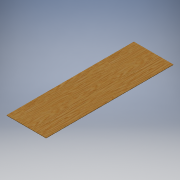
# Autodesk Inventor part: Table top
Saved by Autodesk Inventor 2019.4 (Build 234330000, 330)
## iProperties
Created: 2020-02-27
Part Number: Table top
Material: Plywood, Finish
Document SubType Name: Modeling
Designer: admin
Density: 0.552 g/cm^3
Appearance: Plywood - New
Author: admin
Autodesk Inventor part; units mm, degrees
ref_plane "YZ Plane" through (0, 0, 0) normal (1, 0, 0) x (0, 1, 0)
ref_plane "XZ Plane" through (0, 0, 0) normal (0, 1, 0) x (-1, 0, 0)
ref_plane "XY Plane" through (0, 0, 0) normal (0, 0, 1) x (1, 0, 0)
sketch "Sketch1" plane through (0, 0, 0) normal (0, 1, 0) x (-1, 0, 0)
  line L0 (-225, 725) -> (225, 725)
  line L1 (225, 725) -> (225, -725)
  line L2 (225, -725) -> (-225, -725)
  line L3 (-225, -725) -> (-225, 725)
  line L4 (-225, 725) -> (225, -725) construction
  line L5 (225, 725) -> (-225, -725) construction
  point P0 (0, 0)
  dimension "d0" = 450
  dimension "d1" = 1450
  constraints: 12 end point, 2 midpoint, 2 parallel, 1 horizontal, 1 perpendicular
  measures "d0" distance of L1.end L2.end
  measures "d1" distance of L0.end L1.end
extrude "Extrusion1" add sketch "Sketch1" along normal blind 5
body "Solid1"
